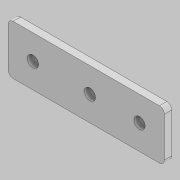
# Autodesk Inventor part: rocker_bogie_mount
Saved by Autodesk Inventor 2021.2 (Build 252289000, 289)
## iProperties
Created: 2021-07-09
Part Number: rocker_bogie_mount
Material: Generic
Document SubType Name: Modeling
Designer: gisen
Density: 1 g/cm^3
Appearance: Default
Author: gisen
Autodesk Inventor part; units mm, degrees
ref_plane "YZ Plane" through (0, 0, 0) normal (1, 0, 0) x (0, 1, 0)
ref_plane "XZ Plane" through (0, 0, 0) normal (0, 1, 0) x (-1, 0, 0)
ref_plane "XY Plane" through (0, 0, 0) normal (0, 0, 1) x (1, 0, 0)
sketch "スケッチ2" plane through (0, 0, 0) normal (0, 0, 1) x (1, 0, 0)
  line L0 (-31.5, 10) -> (31.5, 10)
  line L1 (31.5, 10) -> (31.5, -10)
  line L2 (31.5, -10) -> (-31.5, -10)
  line L3 (-31.5, -10) -> (-31.5, 10)
  line L4 (0, 14) -> (0, -14) construction
  line L5 (-44.1, 0) -> (44.1, 0) construction
  point P0 (0, 0)
  dimension "d1" = 63
  dimension "d2" = 20
  dimension "d3" = 10
  dimension "d4" = 31.5
  constraints: 8 end point, 2 parallel, 1 horizontal, 1 perpendicular
  measures "d1" distance of L1.end L2.end
  measures "d2" distance of L0.end L1.end
  measures "d3" distance between parallel lines of L0 L5
  measures "d4" distance between parallel lines of L4 L3
extrude "押し出し1" add sketch "スケッチ2" along normal blind 3
sketch "スケッチ3" plane through (0, 0, 3) normal (0, 0, 1) x (1, 0, 0)
  line L0 (-31.5, -10) -> (31.5, -10) construction
  line L1 (31.5, -10) -> (31.5, 10) construction
  line L2 (31.5, 10) -> (-31.5, 10) construction
  line L3 (-31.5, 10) -> (-31.5, -10) construction
  line L4 (-44.1, 0) -> (44.1, 0) construction
  point P0 (0, 0)
  point P1 (-21.5, 0)
  point P2 (1.5, 0)
  point P3 (21.5, 0)
  dimension "d7" = 10
  dimension "d8" = 10
  dimension "d9" = 20
  constraints: 3 point on line
  measures "d7" distance from line of point (-21.5, 0) L3
  measures "d8" distance from line of L1 point (21.5, 0)
  measures "d9" distance of point (21.5, 0) point (1.5, 0)
hole "穴1" at (-21.5, 0, 3) at (1.5, 0, 3) at (21.5, 0, 3) direction (0, 0, -1) diameter 4.5 end through all
fillet "フィレット1" radius 2 4 edges at (-31.5, 10, 1.5) (31.5, 10, 1.5) (31.5, -10, 1.5) (-31.5, -10, 1.5)
equation "\"d3\" = 0.5 * d2"
equation "\"d4\" = 0.5 * d1"
